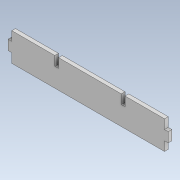
# Autodesk Inventor part: chassis_1_6
Saved by Autodesk Inventor 2022 (Build 260153000, 153)
## iProperties
Created: 2023-04-28
Part Number: chassis_1_6
Material: 一般
Document SubType Name: Modeling
Designer: Johnny Jou
Density: 1 g/cm^3
Appearance: 預設
Author: Johnny Jou
Autodesk Inventor part; units mm, degrees
ref_plane "YZ Plane" through (0, 0, 0) normal (1, 0, 0) x (0, 1, 0)
ref_plane "XZ Plane" through (0, 0, 0) normal (0, 1, 0) x (-1, 0, 0)
ref_plane "XY Plane" through (0, 0, 0) normal (0, 0, 1) x (1, 0, 0)
sketch "草圖1" plane through (0, 0, 0) normal (0, 0, 1) x (1, 0, 0)
  line L0 (0, 0) -> (124, 0)
  line L1 (124, 0) -> (124, -23)
  line L2 (124, -23) -> (0, -23)
  line L3 (0, -23) -> (0, 0)
  line L4 (35, 0) -> (37.95, 0)
  line L5 (37.95, 0) -> (37.95, -7.5)
  line L6 (37.95, -7.5) -> (35, -7.5)
  line L7 (35, -7.5) -> (35, 0)
  line L8 (91.95, 0) -> (89, 0)
  line L9 (89, 0) -> (89, -7.5)
  line L10 (89, -7.5) -> (91.95, -7.5)
  line L11 (91.95, -7.5) -> (91.95, 0)
  line L12 (-3, -7.5) -> (0, -7.5)
  line L13 (0, -7.5) -> (0, -15.5)
  line L14 (0, -15.5) -> (-3, -15.5)
  line L15 (-3, -15.5) -> (-3, -7.5)
  line L16 (124, -7.5) -> (127, -7.5)
  line L17 (127, -7.5) -> (127, -15.5)
  line L18 (127, -15.5) -> (124, -15.5)
  line L19 (124, -15.5) -> (124, -7.5)
  point P0 (124, -15.5)
  point P1 (0, -7.5)
  dimension "d0" = 124
  dimension "d1" = 35
  dimension "d2" = 35
  dimension "d3" = 2.95
  dimension "d4" = 2.95
  dimension "d5" = 8
  dimension "d6" = 3
  dimension "d8" = 8
  dimension "d10" = 15.5
  dimension "d12" = 8
  dimension "d13" = 3
  dimension "d16" = 7.5
  constraints: 40 end point, 10 parallel, 5 horizontal, 5 perpendicular, 5 point on line, 1 collinear
  measures "d0" distance of L1.end L2.end
  measures "d1" distance between parallel lines of L3 L7
  measures "d2" distance between parallel lines of L1 L9
  measures "d3" distance of L5.end L6.end
  measures "d4" distance of L9.end L10.end
  measures "d5" distance of L14.end L12.start
  measures "d6" distance of L13.end L14.end
  measures "d8" distance between parallel lines of L6 L14
  measures "d10" distance between parallel lines of L2 L6
  measures "d12" distance of L16.end L17.end
  measures "d13" distance of L17.end L18.end
  measures "d16" distance of L6.end L4.start
extrude "擠出1" add sketch "草圖1" along normal blind 3 contours L0 L7 L6 L5 L9 L10 L11 L1 L2 L3 | L3 L14 L15 L12 | L1 L16 L17 L18
